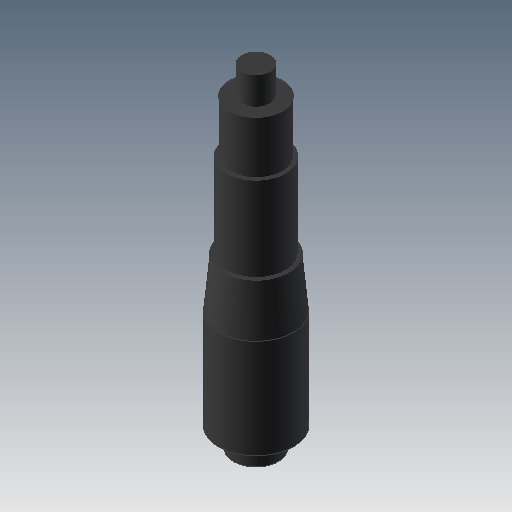
# Autodesk Inventor part: 00_micrometer_xy-stage
Saved by Autodesk Inventor 2019.4 (Build 234330000, 330)
## iProperties
Created: 2021-01-04
Part Number: 00_micrometer_xy-stage
Material: Generic
Document SubType Name: Modeling
Designer: diederichbenedict
Density: 1 g/cm^3
Appearance: Default
Author: diederichbenedict
Autodesk Inventor part; units mm, degrees
ref_plane "YZ Plane" through (0, 0, 0) normal (1, 0, 0) x (0, 1, 0)
ref_plane "XZ Plane" through (0, 0, 0) normal (0, 1, 0) x (-1, 0, 0)
ref_plane "XY Plane" through (0, 0, 0) normal (0, 0, 1) x (1, 0, 0)
sketch "Sketch1" plane through (0, 0, 0) normal (1, 0, 0) x (0, 1, 0)
  line L0 (0, 0) -> (-9.3, 0)
  line L1 (-9.3, 0) -> (-9.3, -4.725)
  line L2 (-9.3, -4.725) -> (0, -4.725)
  line L3 (0, -4.725) -> (0, 0)
  line L4 (0, 0) -> (5, 0)
  line L5 (5, 0) -> (5, -2.5)
  line L6 (5, -2.5) -> (0, -2.5)
  line L7 (0, -2.5) -> (0, 0)
  line L8 (-9.3, 0) -> (-24.3, 0)
  line L9 (-24.3, 0) -> (-24.3, -5.27)
  line L10 (-24.3, -5.27) -> (-9.3, -5.27)
  line L11 (-9.3, -5.27) -> (-9.3, 0)
  line L12 (-24.3, 0) -> (-50.8, 0)
  line L13 (-50.8, 0) -> (-50.8, -6.65)
  line L14 (-50.8, -6.65) -> (-24.3, -6.65)
  line L15 (-24.3, -5.8531) -> (-24.3, 0)
  line L16 (-50.8, 0) -> (-54.4, 0)
  line L17 (-54.4, 0) -> (-54.4, -4)
  line L18 (-54.4, -4) -> (-50.8, -4)
  line L19 (-50.8, -4) -> (-50.8, 0)
  line L20 (-24.3, -5.8531) -> (-33.1623, -6.65)
  dimension "d0" = 9.3
  dimension "d1" = 4.725
  dimension "d2" = 5
  dimension "d3" = 2.5
  dimension "d4" = 15
  dimension "d5" = 26.5
  dimension "d6" = 6.65
  dimension "d7" = 5.27
  dimension "d8" = 3.6
  dimension "d9" = 4
  constraints: 42 end point, 10 parallel, 5 horizontal, 5 perpendicular, 1 point on line
  measures "d0" distance of L2.end L1.end
  measures "d1" distance of L1.end L0.end
  measures "d2" distance of L5.end L6.end
  measures "d3" distance of L4.end L5.end
  measures "d4" distance of L10.end L9.end
  measures "d5" distance of L14.end L13.end
  measures "d6" distance of L13.end L12.end
  measures "d7" distance between parallel lines of L8 L10
  measures "d8" distance of L18.end L17.end
  measures "d9" distance of L17.end L16.end
revolve "Revolution1" add sketch "Sketch1" angle 360 about axis through (0, -9.3, 0) along (0, -1, 0)
body "Solid1"
